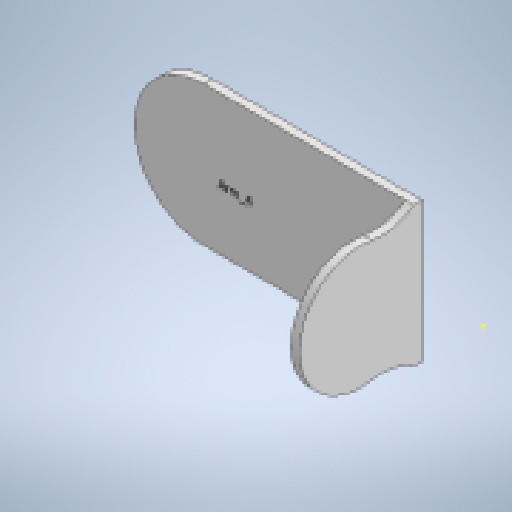
# Autodesk Inventor part: Arm_4
Saved by Autodesk Inventor 2023 (Build 270158000, 158)
## iProperties
Created: 2022-04-08
Part Number: Arm_4
Material: 一般
Document SubType Name: Modeling
Designer: device
Density: 1 g/cm^3
Appearance: 預設
Author: device
Autodesk Inventor part; units mm, degrees
ref_plane "YZ Plane" through (0, 0, 0) normal (1, 0, 0) x (0, 1, 0)
ref_plane "XZ Plane" through (0, 0, 0) normal (0, 1, 0) x (-1, 0, 0)
ref_plane "XY Plane" through (0, 0, 0) normal (0, 0, 1) x (1, 0, 0)
sketch "草圖1" plane through (0, 0, 0) normal (0, 0, 1) x (1, 0, 0)
  line L0 (0, 0) -> (-100, 0) construction
  line L1 (0, 25) -> (-100, 25)
  line L2 (-100, -25) -> (0, -25)
  arc A0 (0, -25) -> (0, 25) centre (0, 0) ccw
  arc A1 (-100, 25) -> (-100, -25) centre (-100, 0) ccw
  circle A2 centre (0, 0) radius 25
  line L3 (-25, 25) -> (-25, -25)
  point P0 (-50, 0)
  point P1 (25, 0)
  point P2 (-125, 0)
  dimension "d0" = 50
  dimension "d1" = 150
  constraints: 10 end point, 6 point on circle, 4 tangent, 2 centre point, 2 point on line, 1 coincident, 1 horizontal, 1 midpoint, 1 parallel, 1 perpendicular, 1 vertical alignment, 2 other
  measures "d0" diameter of A1
  measures "d1" distance of point (25, 0) point (-125, 0)
extrude "擠出1" add sketch "草圖1" along normal mid plane 3 contours L3 L2 A1 L1
sketch "草圖2" plane through (-25, -25, 1.5) normal (1, 0, 0) x (0, 0, -1)
  circle A0 centre (-19, 25) radius 22
  line L0 (3, 50) -> (3, 0) construction
  point P0 (1.5, 25)
  point P1 (3, 25)
  dimension "d4" = 44
  constraints: 1 horizontal alignment, 1 midpoint, 1 vertical, 2 other
extrude "擠出2" add sketch "草圖2" against normal blind 3
fillet "圓角1" radius 20 2 edges at (-26.5, 11.0905, 1.5) (-26.5, -11.0905, 1.5)
sketch "草圖3" plane through (0, 0, 1.5) normal (0, 0, 1) x (1, 0, 0)
  line L0 (-94.9774, -1.6071) -> (-72.1571, -1.6071) construction
  line L1 (-72.1571, -1.6071) -> (-72.1571, -15.4278) construction
  line L2 (-72.1571, -15.4278) -> (-94.9774, -15.4278) construction
  line L3 (-94.9774, -15.4278) -> (-94.9774, -1.6071) construction
  point P0 (0, 0)
  constraints: 2 other
